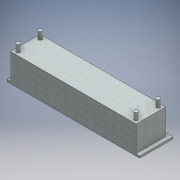
# Autodesk Inventor part: 240531_3Dstorage
Saved by Autodesk Inventor 2016 (Build 200138000, 138)
## iProperties
Created: 2024-05-31
Part Number: 240531_3Dstorage
Material: 일반
Document SubType Name: Modeling
Designer: pc
Density: 1 g/cm^3
Appearance: 목재 - 페인트 흰색
Author: pc
Autodesk Inventor part; units mm, degrees
ref_plane "YZ Plane" through (0, 0, 0) normal (1, 0, 0) x (0, 1, 0)
ref_plane "XZ Plane" through (0, 0, 0) normal (0, 1, 0) x (-1, 0, 0)
ref_plane "XY Plane" through (0, 0, 0) normal (0, 0, 1) x (1, 0, 0)
sketch "스케치1" plane through (0, 0, 0) normal (0, 0, 1) x (1, 0, 0)
  line L0 (900, -225) -> (-900, -225)
  line L1 (-900, -225) -> (-900, 225)
  line L2 (-900, 225) -> (900, 225)
  line L3 (900, 225) -> (900, -225)
  line L4 (900, -225) -> (-900, 225) construction
  line L5 (-900, -225) -> (900, 225) construction
  point P0 (0, 0)
  dimension "d0" = 1800
  dimension "d1" = 450
  constraints: 12 end point, 2 midpoint, 2 parallel, 1 horizontal, 1 perpendicular
  measures "d0" distance of L1.end L2.end
  measures "d1" distance of L0.end L1.end
extrude "돌출1" add sketch "스케치1" along normal blind 30
sketch "스케치2" plane through (0, 0, 30) normal (0, 0, 1) x (1, 0, 0)
  line L0 (-900, -225) -> (900, -225) projected
  line L1 (-850, 175) -> (850, 175)
  line L2 (850, 175) -> (850, -225)
  line L3 (850, -225) -> (-850, -225)
  line L4 (-850, -225) -> (-850, 175)
  line L5 (900, 225) -> (-900, 225) projected
  line L6 (-900, 225) -> (-900, -225) projected
  line L7 (900, -225) -> (900, 225) projected
  point P0 (0, 0)
  dimension "d4" = 50
  dimension "d5" = 50
  dimension "d6" = 50
  constraints: 8 end point, 2 parallel, 1 horizontal, 1 perpendicular, 1 point on line
  measures "d4" distance between parallel lines of L1 L5
  measures "d5" distance between parallel lines of L4 L6
  measures "d6" distance between parallel lines of L7 L2
extrude "돌출2" add sketch "스케치2" along normal blind 350 contours L4 L1 L2 L0
sketch "스케치3" plane through (-850, 175, 30) normal (0, 1, 0) x (1, 0, 0)
  line L0 (0, 0) -> (1700, 0) construction
  line L1 (850, 0) -> (850, -673.9117) construction
  line L2 (30, -30) -> (530, -30)
  line L3 (530, -30) -> (530, -150)
  line L4 (530, -150) -> (30, -150)
  line L5 (30, -150) -> (30, -30)
  line L6 (0, 0) -> (0, -350) projected
  line L7 (1170, -30) -> (1670, -30)
  line L8 (1670, -30) -> (1670, -150)
  line L9 (1670, -150) -> (1170, -150)
  line L10 (1170, -150) -> (1170, -30)
  line L11 (1700, 0) -> (1700, -350) projected
  line L12 (30, -190) -> (530, -190)
  line L13 (530, -190) -> (530, -310)
  line L14 (530, -310) -> (30, -310)
  line L15 (30, -310) -> (30, -190)
  line L16 (1670, -190) -> (1170, -190)
  line L17 (1170, -190) -> (1170, -310)
  line L18 (1170, -310) -> (1670, -310)
  line L19 (1670, -310) -> (1670, -190)
  point P0 (850, 30)
  dimension "d9" = 120
  dimension "d10" = 30
  dimension "d11" = 120
  dimension "d12" = 30
  dimension "d13" = 500
  dimension "d14" = 500
  dimension "d15" = 120
  dimension "d16" = 40
  dimension "d17" = 30
  dimension "d18" = 30
  constraints: 34 end point, 6 parallel, 4 symmetric about line, 3 horizontal, 3 perpendicular, 1 midpoint, 1 vertical
  measures "d9" distance of L4.end L2.start
  measures "d10" distance between parallel lines of L6 L5
  measures "d11" distance of L7.end L8.end
  measures "d12" distance between parallel lines of L11 L8
  measures "d13" distance of L7.start L7.end
  measures "d14" distance of L2.start L2.end
  measures "d15" distance of L12.end L13.end
  measures "d16" distance between parallel lines of L12 L4
  measures "d17" distance between parallel lines of L2 L0
  measures "d18" distance between parallel lines of L0 L7
extrude "돌출3" cut sketch "스케치3" against normal blind 380
sketch "스케치4" plane through (-850, 175, 30) normal (0, 1, 0) x (1, 0, 0)
  line L0 (850, 30) -> (850, -738.9352) construction
  line L1 (1152.4561, -310) -> (547.5439, -310)
  line L2 (547.5439, -310) -> (547.5439, -30)
  line L3 (547.5439, -30) -> (1152.4561, -30)
  line L4 (1152.4561, -30) -> (1152.4561, -310)
  line L5 (1152.4561, -310) -> (547.5439, -30) construction
  line L6 (547.5439, -310) -> (1152.4561, -30) construction
  line L7 (30, -30) -> (530, -30) projected
  line L8 (530, -310) -> (30, -310) projected
  point P0 (850, -170)
  dimension "d21" = 0
  dimension "d22" = 0
  constraints: 14 end point, 2 midpoint, 2 parallel, 1 horizontal, 1 perpendicular, 1 point on line, 1 vertical
  measures "d21" distance between parallel lines of L7 L3
  measures "d22" distance between parallel lines of L8 L1
extrude "돌출4" cut sketch "스케치4" against normal blind 380
sketch "스케치5" plane through (0, 0, 380) normal (0, 0, 1) x (1, 0, 0)
  line L0 (-800, 125) -> (800, 125) construction
  line L1 (800, 125) -> (800, -175) construction
  line L2 (800, -175) -> (-800, -175) construction
  line L3 (-800, -175) -> (-800, 125) construction
  line L4 (850, 175) -> (-850, 175) projected
  line L5 (-850, -225) -> (850, -225) projected
  line L6 (850, -225) -> (850, 175) projected
  line L7 (-850, 175) -> (-850, -225) projected
  circle A0 centre (-800, 125) radius 25
  circle A1 centre (800, 125) radius 25
  circle A2 centre (800, -175) radius 25
  circle A3 centre (-800, -175) radius 25
  point P0 (0, 0)
  dimension "d26" = 50
  dimension "d27" = 50
  dimension "d28" = 50
  dimension "d29" = 50
  dimension "d30" = 50
  dimension "d31" = 50
  dimension "d32" = 50
  dimension "d33" = 50
  constraints: 8 end point, 4 centre point, 4 coincident, 2 parallel, 1 horizontal, 1 perpendicular
  measures "d26" distance between parallel lines of L0 L4
  measures "d27" distance between parallel lines of L2 L5
  measures "d28" distance between parallel lines of L1 L6
  measures "d29" distance between parallel lines of L7 L3
  measures "d30" diameter of A0
  measures "d31" diameter of A1
  measures "d32" diameter of A2
  measures "d33" diameter of A3
extrude "돌출5" add sketch "스케치5" along normal blind 100 contours A0 | A1 | A2 | A3
